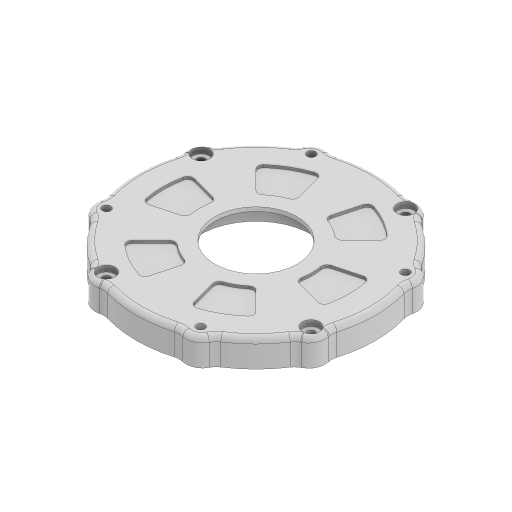
# Autodesk Inventor part: tapa
Saved by Autodesk Inventor 2024.3 (Build 283343000, 343)
## iProperties
Created: 2025-03-05
Part Number: tapa
Material: Generic
Document SubType Name: Modeling
Designer: danie
Density: 1 g/cm^3
Appearance: Default
Author: danie
Autodesk Inventor part; units mm, degrees
ref_plane "YZ Plane" through (0, 0, 0) normal (1, 0, 0) x (0, 1, 0)
ref_plane "XZ Plane" through (0, 0, 0) normal (0, 1, 0) x (-1, 0, 0)
ref_plane "XY Plane" through (0, 0, 0) normal (0, 0, 1) x (1, 0, 0)
sketch "Block1" plane through (0, 0, 0) normal (0, 0, 1) x (1, 0, 0)
  arc A0 (57.7497, -25.9707) -> (44.669, -38.976) centre (82.2635, -63.7077) ccw
  arc A1 (57.7497, -25.9707) -> (59.8142, -23.6885) centre (54.4812, -20.9392) ccw
  arc A2 (66.537, -20.6011) -> (59.8142, -23.6885) centre (65.1472, -26.4379) ccw
  arc A3 (66.537, -20.6011) -> (69.6134, -20.5223) centre (67.9267, -14.7643) ccw
  circle A4 centre (64.557, -25.1528) radius 1.5875
  arc A5 (39.0781, -51.0576) -> (39.1389, -47.9074) centre (33.3201, -49.3709) ccw
  circle A6 centre (43.76, -45.8897) radius 1.5875
  arc A7 (42.307, -41.0612) -> (39.1389, -47.9074) centre (44.9577, -46.444) ccw
  arc A8 (42.307, -41.0612) -> (44.669, -38.976) centre (39.6564, -35.6784) ccw
  arc A9 (94.9136, -20.5223) -> (69.6134, -20.5223) centre (82.2635, -63.7077) ccw
  circle A10 centre (100.0814, -25.2042) radius 1.5875
  arc A11 (104.91, -23.7512) -> (106.9952, -26.1132) centre (110.2927, -21.1006) ccw
  arc A12 (104.91, -23.7512) -> (98.0637, -20.5831) centre (99.5272, -26.4018) ccw
  arc A13 (94.9136, -20.5223) -> (98.0637, -20.5831) centre (96.6003, -14.7643) ccw
  arc A14 (39.0933, -79.3831) -> (39.0417, -76.2328) centre (33.2788, -77.9028) ccw
  arc A15 (39.0781, -51.0576) -> (39.0417, -76.2328) centre (82.2635, -63.7077) ccw
  arc A16 (125.4336, -48.0323) -> (122.2853, -41.1769) centre (119.6191, -46.552) ccw
  arc A17 (119.9293, -39.0849) -> (122.2853, -41.1769) centre (124.9515, -35.8018) ccw
  arc A18 (119.9293, -39.0849) -> (106.9952, -26.1132) centre (82.2635, -63.7077) ccw
  arc A19 (39.0933, -79.3831) -> (42.2417, -86.2385) centre (44.9079, -80.8634) ccw
  circle A20 centre (43.7086, -81.4142) radius 1.5875
  arc A21 (44.5976, -88.3305) -> (57.5318, -101.3021) centre (82.2635, -63.7077) ccw
  arc A22 (44.5976, -88.3305) -> (42.2417, -86.2385) centre (39.5755, -91.6136) ccw
  circle A23 centre (64.4455, -102.2112) radius 1.5875
  arc A24 (59.617, -103.6641) -> (57.5318, -101.3021) centre (54.2342, -106.3147) ccw
  arc A25 (59.617, -103.6641) -> (66.4633, -106.8323) centre (64.9998, -101.0135) ccw
  arc A26 (69.6134, -106.893) -> (66.4633, -106.8323) centre (67.9267, -112.6511) ccw
  arc A27 (125.4336, -48.0323) -> (125.4853, -51.1826) centre (131.2482, -49.5126) ccw
  circle A28 centre (120.8184, -46.0012) radius 1.5875
  arc A29 (125.4164, -76.4679) -> (125.4853, -51.1826) centre (82.2635, -63.7077) ccw
  arc A30 (69.6134, -106.893) -> (94.7886, -106.9295) centre (82.2635, -63.7077) ccw
  arc A31 (125.4164, -76.4679) -> (125.3396, -79.5853) centre (131.1702, -78.1693) ccw
  circle A32 centre (120.767, -81.5256) radius 1.5875
  arc A33 (122.1898, -86.3691) -> (125.3396, -79.5853) centre (119.5091, -81.0013) ccw
  arc A34 (122.1898, -86.3691) -> (119.8579, -88.4394) centre (124.8705, -91.7369) ccw
  arc A35 (97.9063, -106.8696) -> (94.7886, -106.9295) centre (96.4586, -112.6924) ccw
  circle A36 centre (99.97, -102.2626) radius 1.5875
  arc A37 (106.7901, -101.4362) -> (119.8579, -88.4394) centre (82.2635, -63.7077) ccw
  arc A38 (106.7901, -101.4362) -> (104.7072, -103.7568) centre (110.0603, -106.4667) ccw
  arc A39 (97.9063, -106.8696) -> (104.7072, -103.7568) centre (99.354, -101.0469) ccw
  point P0 (82.2553, -63.716)
  point P1 (82.2635, -63.7077)
sketch "Sketch1" plane through (0, 0, 0) normal (0, 1, 0) x (-1, 0, 0)
  circle A0 centre (0, 0) radius 21.1
  circle A1 centre (0, 0) radius 45
  dimension "d0" = 42.2
  dimension "d1" = 90
  constraints: 2 centre point, 2 coincident
  measures "d0" diameter of A0
  measures "d1" diameter of A1
extrude "Extrusion1" add sketch "Sketch1" along normal blind 8
sketch "Sketch2" plane through (0, 8, 0) normal (0, 1, 0) x (1, 0, 0)
  circle A0 centre (0, 0) radius 21.1 projected
  circle A1 centre (0, 0) radius 15
  dimension "d4" = 30
  constraints: 1 centre point, 1 coincident
  measures "d4" diameter of A1
extrude "Extrusion2" add sketch "Sketch2" against normal blind 2
sketch "Sketch5" plane through (0, 8, 0) normal (0, 1, 0) x (1, 0, 0)
  circle A0 centre (0, 0) radius 15 projected
  circle A1 centre (0, 0) radius 45 projected
  line L0 (-35, -35) -> (35, -35)
  line L1 (35, -35) -> (35, 35)
  line L2 (35, 35) -> (-35, 35)
  line L3 (-35, 35) -> (-35, -35)
  line L4 (-35, -35) -> (35, 35) construction
  line L5 (35, -35) -> (-35, 35) construction
  line L6 (-30, -30) -> (30, -30)
  line L7 (30, -30) -> (30, 30)
  line L8 (30, 30) -> (-30, 30)
  line L9 (-30, 30) -> (-30, -30)
  line L10 (-30, -30) -> (30, 30) construction
  line L11 (30, -30) -> (-30, 30) construction
  circle A2 centre (-30, 30) radius 1.5875
  circle A3 centre (30, 30) radius 1.5875
  circle A4 centre (-30, -30) radius 1.5875
  circle A5 centre (30, -30) radius 1.5875
  point P0 (35, -28.2843)
  point P1 (28.2843, -35)
  point P2 (-35, -28.2843)
  point P3 (-28.2843, -35)
  point P4 (28.2843, 35)
  point P5 (35, 28.2843)
  point P6 (-35, 28.2843)
  point P7 (-28.2843, 35)
  dimension "d24" = 70
  dimension "d25" = 70
  dimension "d26" = 60
  dimension "d27" = 3.175
  dimension "d30" = 60
  dimension "d33" = 60
  constraints: 24 end point, 4 centre point, 4 midpoint, 4 parallel, 3 horizontal, 2 perpendicular, 1 coincident, 1 point on line, 1 vertical, 6 other
  measures "d24" distance between parallel lines of L1 L3
  measures "d25" distance between parallel lines of L0 L2
  measures "d26" distance of L6.end L7.end
  measures "d27" diameter of A2
  measures "d30" distance of A2.centre A3.centre
  measures "d33" distance of A2.centre A4.centre
sketch "Sketch7" plane through (0, 8, 0) normal (0, 1, 0) x (1, 0, 0)
  circle A0 centre (0, 0) radius 15 projected
  circle A1 centre (0, 0) radius 45 projected
  circle A2 centre (0, 0) radius 12.6501
  arc A3 (-24.5138, 37.7369) -> (-37.5945, 24.7317) centre (0, 0) ccw
  arc A4 (-24.5138, 37.7369) -> (-22.4493, 40.0191) centre (-27.7823, 42.7685) ccw
  arc A5 (-15.7265, 43.1066) -> (-22.4493, 40.0191) centre (-17.1163, 37.2697) ccw
  arc A6 (-15.7265, 43.1066) -> (-12.6501, 43.1854) centre (-14.3368, 48.9434) ccw
  circle A7 centre (-17.7065, 38.5549) radius 1.5875
  arc A8 (-43.1854, 12.6501) -> (-43.1246, 15.8002) centre (-48.9434, 14.3368) ccw
  circle A9 centre (-38.5035, 17.8179) radius 1.5875
  arc A10 (-39.9564, 22.6465) -> (-43.1246, 15.8002) centre (-37.3058, 17.2637) ccw
  arc A11 (-39.9564, 22.6465) -> (-37.5945, 24.7317) centre (-42.607, 28.0293) ccw
  arc A12 (12.6501, 43.1854) -> (-12.6501, 43.1854) centre (0, 0) ccw
  circle A13 centre (17.8179, 38.5035) radius 1.5875
  arc A14 (22.6465, 39.9564) -> (24.7317, 37.5945) centre (28.0293, 42.607) ccw
  arc A15 (22.6465, 39.9564) -> (15.8002, 43.1246) centre (17.2637, 37.3058) ccw
  arc A16 (12.6501, 43.1854) -> (15.8002, 43.1246) centre (14.3368, 48.9434) ccw
  arc A17 (-43.1702, -15.6754) -> (-43.2218, -12.5251) centre (-48.9847, -14.1951) ccw
  arc A18 (-43.1854, 12.6501) -> (-43.2218, -12.5251) centre (0, 0) ccw
  arc A19 (43.1702, 15.6754) -> (40.0218, 22.5308) centre (37.3556, 17.1557) ccw
  arc A20 (37.6659, 24.6228) -> (40.0218, 22.5308) centre (42.688, 27.9059) ccw
  arc A21 (37.6659, 24.6228) -> (24.7317, 37.5945) centre (0, 0) ccw
  arc A22 (-43.1702, -15.6754) -> (-40.0218, -22.5308) centre (-37.3556, -17.1557) ccw
  circle A23 centre (-38.5549, -17.7065) radius 1.5875
  arc A24 (-37.6659, -24.6228) -> (-24.7317, -37.5945) centre (0, 0) ccw
  arc A25 (-37.6659, -24.6228) -> (-40.0218, -22.5308) centre (-42.688, -27.9059) ccw
  circle A26 centre (-17.8179, -38.5035) radius 1.5875
  arc A27 (-22.6465, -39.9564) -> (-24.7317, -37.5945) centre (-28.0293, -42.607) ccw
  arc A28 (-22.6465, -39.9564) -> (-15.8002, -43.1246) centre (-17.2637, -37.3058) ccw
  arc A29 (-12.6501, -43.1854) -> (-15.8002, -43.1246) centre (-14.3368, -48.9434) ccw
  arc A30 (43.1702, 15.6754) -> (43.2218, 12.5251) centre (48.9847, 14.1951) ccw
  circle A31 centre (38.5549, 17.7065) radius 1.5875
  arc A32 (43.1529, -12.7603) -> (43.2218, 12.5251) centre (0, 0) ccw
  arc A33 (-12.6501, -43.1854) -> (12.5251, -43.2218) centre (0, 0) ccw
  arc A34 (43.1529, -12.7603) -> (43.0761, -15.8776) centre (48.9067, -14.4616) ccw
  circle A35 centre (38.5035, -17.8179) radius 1.5875
  arc A36 (39.9263, -22.6614) -> (43.0761, -15.8776) centre (37.2456, -17.2936) ccw
  arc A37 (39.9263, -22.6614) -> (37.5945, -24.7317) centre (42.607, -28.0293) ccw
  arc A38 (15.6428, -43.162) -> (12.5251, -43.2218) centre (14.1951, -48.9847) ccw
  circle A39 centre (17.7065, -38.5549) radius 1.5875
  arc A40 (24.5266, -37.7286) -> (37.5945, -24.7317) centre (0, 0) ccw
  arc A41 (24.5266, -37.7286) -> (22.4437, -40.0491) centre (27.7968, -42.759) ccw
  arc A42 (15.6428, -43.162) -> (22.4437, -40.0491) centre (17.0905, -37.3392) ccw
  point P0 (-12.6501, -43.1854)
  point P1 (24.5266, -37.7286)
  point P2 (12.5251, -43.2218)
  point P3 (43.1529, -12.7603)
  point P4 (37.5945, -24.7317)
  point P5 (37.6659, 24.6228)
  point P6 (43.2218, 12.5251)
  point P7 (12.6501, 43.1854)
  point P8 (24.7317, 37.5945)
  point P9 (-24.5138, 37.7369)
  point P10 (-12.6501, 43.1854)
  point P11 (-43.1854, 12.6501)
  point P12 (-37.5945, 24.7317)
  point P13 (-37.6659, -24.6228)
  point P14 (-43.2218, -12.5251)
  constraints: 1 centre point, 1 concentric, 1 other
extrude "Extrusion6" add sketch "Sketch7" against normal up to surface (8 mm away) contours A1 A20 A19 A30 | A34 A36 A37 A1 | A1 A16 A15 A14 | A41 A42 A38 A1 | A1 A4 A5 A6 | A29 A28 A27 A1 | A1 A8 A10 A11 | A25 A22 A17 A1
extrude "Extrusion7" cut sketch "Sketch7" against normal blind 10 contours A7 | A9 | A13 | A23 | A26 | A31 | A35 | A39
sketch "Sketch3" plane through (0, 8, 0) normal (0, 1, 0) x (1, 0, 0)
  circle A0 centre (0, 0) radius 15 projected
  circle A1 centre (0, 0) radius 45 projected
  circle A2 centre (0, 0) radius 41
  circle A3 centre (-41, 0) radius 1.75
  dimension "d7" = 82
  dimension "d8" = 3.5
  constraints: 1 centre point, 1 coincident, 1 horizontal alignment, 2 other
  measures "d8" diameter of A3
sketch "Sketch4" plane through (0, 8, 0) normal (0, 1, 0) x (1, 0, 0)
  circle A0 centre (0, 0) radius 15 projected
  circle A1 centre (-41, 0) radius 1.75 projected
  circle A2 centre (-20.5, -35.507) radius 1.75 projected
  circle A3 centre (20.5, -35.507) radius 1.75 projected
  circle A4 centre (41, 0) radius 1.75 projected
  circle A5 centre (20.5, 35.507) radius 1.75 projected
  circle A6 centre (-20.5, 35.507) radius 1.75 projected
  circle A7 centre (0, 0) radius 43 projected
move faces "Move1" translate (0, 2.2, 0) faces at (32.4873, 8, -6.8478)
sketch "Sketch8" plane through (0, 0, 0) normal (0, -1, 0) x (1, 0, 0)
  circle A0 centre (17.7065, 38.5549) radius 1.5875 projected
  circle A1 centre (-17.7065, -38.5549) radius 1.5875 projected
  circle A2 centre (17.8179, -38.5035) radius 1.5875 projected
  circle A3 centre (-17.8179, 38.5035) radius 1.5875 projected
  circle A4 centre (38.5035, 17.8179) radius 1.5875 projected
  circle A5 centre (-38.5035, -17.8179) radius 1.5875 projected
  circle A6 centre (38.5549, -17.7065) radius 1.5875 projected
  circle A7 centre (-38.5549, 17.7065) radius 1.5875 projected
  arc A8 (-43.2218, 12.5251) -> (-43.1854, -12.6501) centre (0, 0) ccw projected
  arc A9 (-43.1246, -15.8002) -> (-43.1854, -12.6501) centre (-48.9434, -14.3368) ccw projected
  arc A10 (-43.1246, -15.8002) -> (-39.9564, -22.6465) centre (-37.3058, -17.2637) ccw projected
  arc A11 (-37.5945, -24.7317) -> (-39.9564, -22.6465) centre (-42.607, -28.0293) ccw projected
  arc A12 (-37.5945, -24.7317) -> (-24.5138, -37.7369) centre (0, 0) ccw projected
  arc A13 (-22.4493, -40.0191) -> (-24.5138, -37.7369) centre (-27.7823, -42.7685) ccw projected
  arc A14 (-22.4493, -40.0191) -> (-15.7265, -43.1066) centre (-17.1163, -37.2697) ccw projected
  arc A15 (-12.6501, -43.1854) -> (-15.7265, -43.1066) centre (-14.3368, -48.9434) ccw projected
  arc A16 (-12.6501, -43.1854) -> (12.6501, -43.1854) centre (0, 0) ccw projected
  arc A17 (15.8002, -43.1246) -> (12.6501, -43.1854) centre (14.3368, -48.9434) ccw projected
  arc A18 (15.8002, -43.1246) -> (22.6465, -39.9564) centre (17.2637, -37.3058) ccw projected
  arc A19 (24.7317, -37.5945) -> (22.6465, -39.9564) centre (28.0293, -42.607) ccw projected
  arc A20 (24.7317, -37.5945) -> (37.6659, -24.6228) centre (0, 0) ccw projected
  arc A21 (40.0218, -22.5308) -> (37.6659, -24.6228) centre (42.688, -27.9059) ccw projected
  arc A22 (40.0218, -22.5308) -> (43.1702, -15.6754) centre (37.3556, -17.1557) ccw projected
  arc A23 (43.2218, -12.5251) -> (43.1702, -15.6754) centre (48.9847, -14.1951) ccw projected
  arc A24 (43.2218, -12.5251) -> (43.1529, 12.7603) centre (0, 0) ccw projected
  arc A25 (43.0761, 15.8776) -> (43.1529, 12.7603) centre (48.9067, 14.4616) ccw projected
  arc A26 (43.0761, 15.8776) -> (39.9263, 22.6614) centre (37.2456, 17.2936) ccw projected
  arc A27 (37.5945, 24.7317) -> (39.9263, 22.6614) centre (42.607, 28.0293) ccw projected
  arc A28 (37.5945, 24.7317) -> (24.5266, 37.7286) centre (0, 0) ccw projected
  arc A29 (22.4437, 40.0491) -> (24.5266, 37.7286) centre (27.7968, 42.759) ccw projected
  arc A30 (22.4437, 40.0491) -> (15.6428, 43.162) centre (17.0905, 37.3392) ccw projected
  arc A31 (12.5251, 43.2218) -> (15.6428, 43.162) centre (14.1951, 48.9847) ccw projected
  arc A32 (12.5251, 43.2218) -> (-12.6501, 43.1854) centre (0, 0) ccw projected
  arc A33 (-15.8002, 43.1246) -> (-12.6501, 43.1854) centre (-14.3368, 48.9434) ccw projected
  arc A34 (-15.8002, 43.1246) -> (-22.6465, 39.9564) centre (-17.2637, 37.3058) ccw projected
  arc A35 (-24.7317, 37.5945) -> (-22.6465, 39.9564) centre (-28.0293, 42.607) ccw projected
  arc A36 (-24.7317, 37.5945) -> (-37.6659, 24.6228) centre (0, 0) ccw projected
  arc A37 (-40.0218, 22.5308) -> (-37.6659, 24.6228) centre (-42.688, 27.9059) ccw projected
  arc A38 (-40.0218, 22.5308) -> (-43.1702, 15.6754) centre (-37.3556, 17.1557) ccw projected
  arc A39 (-43.2218, 12.5251) -> (-43.1702, 15.6754) centre (-48.9847, 14.1951) ccw projected
  circle A40 centre (0, 0) radius 21.1 projected
  circle A41 centre (0, 0) radius 31.25
  dimension "d52" = 62.5
  constraints: 1 centre point, 1 coincident
  measures "d52" diameter of A41
extrude "Extrusion8" cut sketch "Sketch8" against normal blind 1.5 contours A41
move faces "Move2" translate (0, 2.7, 0) faces at (-18.717, 6, 2.8798)
sketch "Sketch9" plane through (0, 10.2, 0) normal (0, 1, 0) x (1, 0, 0)
  circle A0 centre (17.7065, -38.5549) radius 1.5875 projected
  circle A1 centre (-17.7065, 38.5549) radius 1.5875 projected
  circle A2 centre (17.8179, 38.5035) radius 1.5875 projected
  circle A3 centre (-17.8179, -38.5035) radius 1.5875 projected
  circle A4 centre (38.5035, -17.8179) radius 1.5875 projected
  circle A5 centre (-38.5035, 17.8179) radius 1.5875 projected
  circle A6 centre (38.5549, 17.7065) radius 1.5875 projected
  circle A7 centre (-38.5549, -17.7065) radius 1.5875 projected
  circle A8 centre (0, 0) radius 15 projected
  arc A9 (-43.1854, 12.6501) -> (-43.2218, -12.5251) centre (0, 0) ccw projected
  arc A10 (-43.1702, -15.6754) -> (-43.2218, -12.5251) centre (-48.9847, -14.1951) ccw projected
  arc A11 (-43.1702, -15.6754) -> (-40.0218, -22.5308) centre (-37.3556, -17.1557) ccw projected
  arc A12 (-37.6659, -24.6228) -> (-40.0218, -22.5308) centre (-42.688, -27.9059) ccw projected
  arc A13 (-37.6659, -24.6228) -> (-24.7317, -37.5945) centre (0, 0) ccw projected
  arc A14 (-22.6465, -39.9564) -> (-24.7317, -37.5945) centre (-28.0293, -42.607) ccw projected
  arc A15 (-22.6465, -39.9564) -> (-15.8002, -43.1246) centre (-17.2637, -37.3058) ccw projected
  arc A16 (-12.6501, -43.1854) -> (-15.8002, -43.1246) centre (-14.3368, -48.9434) ccw projected
  arc A17 (-12.6501, -43.1854) -> (12.5251, -43.2218) centre (0, 0) ccw projected
  arc A18 (15.6428, -43.162) -> (12.5251, -43.2218) centre (14.1951, -48.9847) ccw projected
  arc A19 (15.6428, -43.162) -> (22.4437, -40.0491) centre (17.0905, -37.3392) ccw projected
  arc A20 (24.5266, -37.7286) -> (22.4437, -40.0491) centre (27.7968, -42.759) ccw projected
  arc A21 (24.5266, -37.7286) -> (37.5945, -24.7317) centre (0, 0) ccw projected
  arc A22 (39.9263, -22.6614) -> (37.5945, -24.7317) centre (42.607, -28.0293) ccw projected
  arc A23 (39.9263, -22.6614) -> (43.0761, -15.8776) centre (37.2456, -17.2936) ccw projected
  arc A24 (43.1529, -12.7603) -> (43.0761, -15.8776) centre (48.9067, -14.4616) ccw projected
  arc A25 (43.1529, -12.7603) -> (43.2218, 12.5251) centre (0, 0) ccw projected
  arc A26 (43.1702, 15.6754) -> (43.2218, 12.5251) centre (48.9847, 14.1951) ccw projected
  arc A27 (43.1702, 15.6754) -> (40.0218, 22.5308) centre (37.3556, 17.1557) ccw projected
  arc A28 (37.6659, 24.6228) -> (40.0218, 22.5308) centre (42.688, 27.9059) ccw projected
  arc A29 (37.6659, 24.6228) -> (24.7317, 37.5945) centre (0, 0) ccw projected
  arc A30 (22.6465, 39.9564) -> (24.7317, 37.5945) centre (28.0293, 42.607) ccw projected
  arc A31 (22.6465, 39.9564) -> (15.8002, 43.1246) centre (17.2637, 37.3058) ccw projected
  arc A32 (12.6501, 43.1854) -> (15.8002, 43.1246) centre (14.3368, 48.9434) ccw projected
  arc A33 (12.6501, 43.1854) -> (-12.6501, 43.1854) centre (0, 0) ccw projected
  arc A34 (-15.7265, 43.1066) -> (-12.6501, 43.1854) centre (-14.3368, 48.9434) ccw projected
  arc A35 (-15.7265, 43.1066) -> (-22.4493, 40.0191) centre (-17.1163, 37.2697) ccw projected
  arc A36 (-24.5138, 37.7369) -> (-22.4493, 40.0191) centre (-27.7823, 42.7685) ccw projected
  arc A37 (-24.5138, 37.7369) -> (-37.5945, 24.7317) centre (0, 0) ccw projected
  arc A38 (-39.9564, 22.6465) -> (-37.5945, 24.7317) centre (-42.607, 28.0293) ccw projected
  arc A39 (-39.9564, 22.6465) -> (-43.1246, 15.8002) centre (-37.3058, 17.2637) ccw projected
  arc A40 (-43.1854, 12.6501) -> (-43.1246, 15.8002) centre (-48.9434, 14.3368) ccw projected
  circle A41 centre (0, 0) radius 15.5
  dimension "d58" = 31
  constraints: 1 centre point, 1 coincident
  measures "d58" diameter of A41
extrude "Extrusion9" cut sketch "Sketch9" against normal up to surface (1.5 mm away) contours A41
sketch "Sketch10" plane through (0, 10.2, 0) normal (0, 1, 0) x (1, 0, 0)
  circle A0 centre (0, 0) radius 15.5 projected
  circle A1 centre (17.7065, -38.5549) radius 1.5875 projected
  circle A2 centre (-17.7065, 38.5549) radius 1.5875 projected
  circle A3 centre (17.8179, 38.5035) radius 1.5875 projected
  circle A4 centre (-17.8179, -38.5035) radius 1.5875 projected
  circle A5 centre (38.5035, -17.8179) radius 1.5875 projected
  circle A6 centre (-38.5035, 17.8179) radius 1.5875 projected
  circle A7 centre (38.5549, 17.7065) radius 1.5875 projected
  circle A8 centre (-38.5549, -17.7065) radius 1.5875 projected
  arc A9 (-43.1854, 12.6501) -> (-43.2218, -12.5251) centre (0, 0) ccw projected
  arc A10 (-43.1702, -15.6754) -> (-43.2218, -12.5251) centre (-48.9847, -14.1951) ccw projected
  arc A11 (-43.1702, -15.6754) -> (-40.0218, -22.5308) centre (-37.3556, -17.1557) ccw projected
  arc A12 (-37.6659, -24.6228) -> (-40.0218, -22.5308) centre (-42.688, -27.9059) ccw projected
  arc A13 (-37.6659, -24.6228) -> (-24.7317, -37.5945) centre (0, 0) ccw projected
  arc A14 (-22.6465, -39.9564) -> (-24.7317, -37.5945) centre (-28.0293, -42.607) ccw projected
  arc A15 (-22.6465, -39.9564) -> (-15.8002, -43.1246) centre (-17.2637, -37.3058) ccw projected
  arc A16 (-12.6501, -43.1854) -> (-15.8002, -43.1246) centre (-14.3368, -48.9434) ccw projected
  arc A17 (-12.6501, -43.1854) -> (12.5251, -43.2218) centre (0, 0) ccw projected
  arc A18 (15.6428, -43.162) -> (12.5251, -43.2218) centre (14.1951, -48.9847) ccw projected
  arc A19 (15.6428, -43.162) -> (22.4437, -40.0491) centre (17.0905, -37.3392) ccw projected
  arc A20 (24.5266, -37.7286) -> (22.4437, -40.0491) centre (27.7968, -42.759) ccw projected
  arc A21 (24.5266, -37.7286) -> (37.5945, -24.7317) centre (0, 0) ccw projected
  arc A22 (39.9263, -22.6614) -> (37.5945, -24.7317) centre (42.607, -28.0293) ccw projected
  arc A23 (39.9263, -22.6614) -> (43.0761, -15.8776) centre (37.2456, -17.2936) ccw projected
  arc A24 (43.1529, -12.7603) -> (43.0761, -15.8776) centre (48.9067, -14.4616) ccw projected
  arc A25 (43.1529, -12.7603) -> (43.2218, 12.5251) centre (0, 0) ccw projected
  arc A26 (43.1702, 15.6754) -> (43.2218, 12.5251) centre (48.9847, 14.1951) ccw projected
  arc A27 (43.1702, 15.6754) -> (40.0218, 22.5308) centre (37.3556, 17.1557) ccw projected
  arc A28 (37.6659, 24.6228) -> (40.0218, 22.5308) centre (42.688, 27.9059) ccw projected
  arc A29 (37.6659, 24.6228) -> (24.7317, 37.5945) centre (0, 0) ccw projected
  arc A30 (22.6465, 39.9564) -> (24.7317, 37.5945) centre (28.0293, 42.607) ccw projected
  arc A31 (22.6465, 39.9564) -> (15.8002, 43.1246) centre (17.2637, 37.3058) ccw projected
  arc A32 (12.6501, 43.1854) -> (15.8002, 43.1246) centre (14.3368, 48.9434) ccw projected
  arc A33 (12.6501, 43.1854) -> (-12.6501, 43.1854) centre (0, 0) ccw projected
  arc A34 (-15.7265, 43.1066) -> (-12.6501, 43.1854) centre (-14.3368, 48.9434) ccw projected
  arc A35 (-15.7265, 43.1066) -> (-22.4493, 40.0191) centre (-17.1163, 37.2697) ccw projected
  arc A36 (-24.5138, 37.7369) -> (-22.4493, 40.0191) centre (-27.7823, 42.7685) ccw projected
  arc A37 (-24.5138, 37.7369) -> (-37.5945, 24.7317) centre (0, 0) ccw projected
  arc A38 (-39.9564, 22.6465) -> (-37.5945, 24.7317) centre (-42.607, 28.0293) ccw projected
  arc A39 (-39.9564, 22.6465) -> (-43.1246, 15.8002) centre (-37.3058, 17.2637) ccw projected
  arc A40 (-43.1854, 12.6501) -> (-43.1246, 15.8002) centre (-48.9434, 14.3368) ccw projected
hole "Hole2" at (-38.5035, 10.2, -17.8179) at (17.8179, 10.2, -38.5035) at (-17.8179, 10.2, 38.5035) at (38.5035, 10.2, 17.8179) direction (0, -1, 0) diameter 3.175 depth 15 tip angle 118 counterbore diameter 6.5 counterbore depth 2.2
fillet "Fillet1" radius 2 32 edges at (31.8658, 10.2, -31.7737) (23.5313, 10.2, -38.6361) (19.7835, 10.2, -42.7511) (14.2211, 10.2, -42.9445) (0, 10.2, -45) (-14.1832, 10.2, -42.9454) (-19.6203, 10.2, -42.7222) (-23.3327, 10.2, -38.7434) (-31.7276, 10.2, -31.9117) (-38.6361, 10.2, -23.5313) (-42.7511, 10.2, -19.7835) (-42.9445, 10.2, -14.2211) (-45, 10.2, -0.0651) (-42.9855, 10.2, 14.0968) (-42.8081, 10.2, 19.6598) (-38.704, 10.2, 23.4194) (-31.8658, 10.2, 31.7737) (-23.5313, 10.2, 38.6361) (-19.7835, 10.2, 42.7511) (-14.2211, 10.2, 42.9445) (-0.0651, 10.2, 45) (14.08, 10.2, 42.9858) (19.5876, 10.2, 42.7949) (23.3318, 10.2, 38.7512) (31.7331, 10.2, 31.9063) (38.6235, 10.2, 23.5424) (42.6876, 10.2, 19.8204) (42.9085, 10.2, 14.3138) (44.9998, 10.2, 0.1225) (42.9855, 10.2, -14.0968) (42.8081, 10.2, -19.6598) (38.704, 10.2, -23.4194)
sketch "Sketch11" plane through (0, 10.2, 0) normal (0, 1, 0) x (1, 0, 0)
  circle A0 centre (0, 0) radius 21.1 projected
  circle A1 centre (-38.5549, -17.7065) radius 1.5875 projected
  circle A2 centre (38.5549, 17.7065) radius 1.5875 projected
  circle A3 centre (-17.7065, 38.5549) radius 1.5875 projected
  circle A4 centre (17.7065, -38.5549) radius 1.5875 projected
  circle A5 centre (0, 0) radius 15.5 projected
  arc A6 (12.0879, 41.266) -> (15.8463, 41.0871) centre (14.3368, 48.9434) ccw projected
  arc A7 (12.0879, 41.266) -> (-12.0879, 41.266) centre (0, 0) ccw projected
  arc A8 (-16.1898, 41.161) -> (-12.0879, 41.266) centre (-14.3368, 48.9434) ccw projected
  arc A9 (-16.1898, 41.161) -> (-20.6716, 39.1027) centre (-17.1163, 37.2697) ccw projected
  arc A10 (-23.4243, 36.0597) -> (-20.6716, 39.1027) centre (-27.7823, 42.7685) ccw projected
  arc A11 (-23.4243, 36.0597) -> (-35.9236, 23.6325) centre (0, 0) ccw projected
  arc A12 (-38.6727, 21.0635) -> (-35.9236, 23.6325) centre (-42.607, 28.0293) ccw projected
  arc A13 (-41.0871, 15.8463) -> (-38.6727, 21.0635) centre (-38.5035, 17.8179) ccw projected
  arc A14 (-41.266, 12.0879) -> (-41.0871, 15.8463) centre (-48.9434, 14.3368) ccw projected
  arc A15 (-41.266, 12.0879) -> (-41.3008, -11.9684) centre (0, 0) ccw projected
  arc A16 (-41.232, -16.1688) -> (-41.3008, -11.9684) centre (-48.9847, -14.1951) ccw projected
  arc A17 (-41.232, -16.1688) -> (-39.1331, -20.7391) centre (-37.3556, -17.1557) ccw projected
  arc A18 (-35.9918, -23.5285) -> (-39.1331, -20.7391) centre (-42.688, -27.9059) ccw projected
  arc A19 (-35.9918, -23.5285) -> (-23.6325, -35.9236) centre (0, 0) ccw projected
  arc A20 (-21.0635, -38.6727) -> (-23.6325, -35.9236) centre (-28.0293, -42.607) ccw projected
  arc A21 (-15.8463, -41.0871) -> (-21.0635, -38.6727) centre (-17.8179, -38.5035) ccw projected
  arc A22 (-12.0879, -41.266) -> (-15.8463, -41.0871) centre (-14.3368, -48.9434) ccw projected
  arc A23 (-12.0879, -41.266) -> (11.9684, -41.3008) centre (0, 0) ccw projected
  arc A24 (16.1254, -41.221) -> (11.9684, -41.3008) centre (14.1951, -48.9847) ccw projected
  arc A25 (16.1254, -41.221) -> (20.6593, -39.1458) centre (17.0905, -37.3392) ccw projected
  arc A26 (23.4366, -36.0517) -> (20.6593, -39.1458) centre (27.7968, -42.759) ccw projected
  arc A27 (23.4366, -36.0517) -> (35.9236, -23.6325) centre (0, 0) ccw projected
  arc A28 (38.6727, -21.0635) -> (35.9236, -23.6325) centre (42.607, -28.0293) ccw projected
  arc A29 (41.0112, -15.7505) -> (38.6727, -21.0635) centre (38.5035, -17.8179) ccw projected
  arc A30 (41.235, -12.1931) -> (41.0112, -15.7505) centre (48.9067, -14.4616) ccw projected
  arc A31 (41.235, -12.1931) -> (41.3008, 11.9684) centre (0, 0) ccw projected
  arc A32 (41.232, 16.1688) -> (41.3008, 11.9684) centre (48.9847, 14.1951) ccw projected
  arc A33 (41.232, 16.1688) -> (39.1331, 20.7391) centre (37.3556, 17.1557) ccw projected
  arc A34 (35.9918, 23.5285) -> (39.1331, 20.7391) centre (42.688, 27.9059) ccw projected
  arc A35 (35.9918, 23.5285) -> (23.6325, 35.9236) centre (0, 0) ccw projected
  arc A36 (21.0635, 38.6727) -> (23.6325, 35.9236) centre (28.0293, 42.607) ccw projected
  arc A37 (15.8463, 41.0871) -> (21.0635, 38.6727) centre (17.8179, 38.5035) ccw projected
  circle A38 centre (0, 0) radius 35
  line L0 (-21.1, 0) -> (-35, 0)
  line L1 (0, 0) -> (-33.8074, 9.0587)
  line L2 (0, 0) -> (-33.8074, -9.0587)
  point P0 (-20.381, -5.4611)
  point P1 (-20.381, 5.4611)
  dimension "d69" = 70
  dimension "d70" = 15
  dimension "d71" = 15
  dimension "d43" = 42.4264
  dimension "d44" = 45
  constraints: 6 end point, 3 point on circle, 1 centre point, 1 coincident, 1 horizontal, 2 other
  measures "d69" diameter of A38
  measures "d70" angle of L0 L2
  measures "d71" angle of L1 L0
extrude "Extrusion10" cut sketch "Sketch11" against normal blind 1 contours A0 L0 A38 L1 | L2 A38 L0 A0
fillet "Fillet3" radius 2 4 edges at (-20.381, 9.7, 5.4611) (-20.381, 9.7, -5.4611) (-33.8074, 9.7, 9.0587) (-33.8074, 9.7, -9.0587)
pattern_circular "Circular Pattern3" count 6 over 360 about axis through (0, 10.2, 0) along (0, -1, 0) of "Extrusion10", "Fillet3"
body "Solid1"
